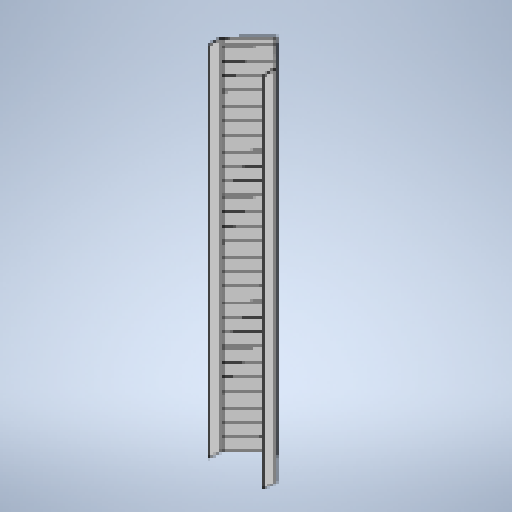
# Autodesk Inventor part: DSB-514 roof 4
Saved by Autodesk Inventor 2025 (Build 290162010, 162A)
## iProperties
Created: 2024-07-24
Part Number: DSB-514 roof 4
Material: Stainless Steel
Document SubType Name: Sheet Metal
Designer: admin
Density: 8 g/cm^3
Flat Pattern Width: 7.85084 cm
Flat Pattern Length: 27.5 cm
Flat Pattern Area: 215.898 cm^2
Sheet Metal Rule: Default
Sheet Metal Width: 78,508 mm
Sheet Metal Length: 275,000 mm
Sheet Metal Area: 21589,801 mm^2
Appearance: Default
Author: admin
Autodesk Inventor part; units mm, degrees
note: some values were not read from the file. Chosen so that the rebuilt part matches the saved one: flange form of "Plate1".
ref_plane "YZ Plane" through (0, 0, 0) normal (1, 0, 0) x (0, 1, 0)
ref_plane "XZ Plane" through (0, 0, 0) normal (0, 1, 0) x (-1, 0, 0)
ref_plane "XY Plane" through (0, 0, 0) normal (0, 0, 1) x (1, 0, 0)
sketch "Sketch3" plane through (0, 0, 0) normal (0, 0, 1) x (1, 0, 0)
  line L0 (-21, -10) -> (-21, -0.404026)
  line L1 (-21, 0) -> (-20.71934, 0.290632) construction
  line L2 (0, 21.746137) -> (0.71934, 21.001238) construction
  line L3 (21, 0) -> (21, -0.404026) construction
  line L4 (0, 21.746137) -> (0, 0) construction
  arc A0 (0.71934, 21.001238) -> (-0.71934, 21.001238) centre (0, 20.30658) ccw
  arc A1 (-20.71934, 0.290632) -> (-21, -0.404026) centre (-20, -0.404026) ccw
  arc A2 (21, -0.404026) -> (20.71934, 0.290632) centre (20, -0.404026) ccw
  line L5 (20.71934, 0.290632) -> (21, 0) construction
  line L6 (21, -0.404026) -> (21, -10)
  line L7 (-20.71934, 0.290632) -> (-0.71934, 21.001238)
  line L8 (-21, -0.404026) -> (-21, 0) construction
  line L9 (0.71934, 21.001238) -> (20.71934, 0.290632)
  line L10 (-0.71934, 21.001238) -> (0, 21.746137) construction
  dimension "d15" = 10
  dimension "d18" = 1
  dimension "d19" = 1
  dimension "d20" = 1
  dimension "d32" = 42
  dimension "d33" = 88
  measures "d15" distance of L3.start L6.end
  measures "d18" radius of A0
  measures "d19" radius of A1
  measures "d20" radius of A2
  measures "d32" distance between parallel lines of L6 L0
  measures "d33" angle of L9 L7
contour flange "Contour Flange1" sketch "Sketch3" thickness 0.8 bend radius 0.8 width 275 along (0, 0, -1) mid plane no both sides no wall seen from (-21, -5.202013, 0) lies toward (1, 0, 0) curves L0 A1 L7 A0 L9 A2 L6
bend "Bend1"
corner "Corner1"
sketch "Sketch5" plane through (20.71934, 0.290632, 0) normal (0.7193398, 0.6946584, 0) x (-0.6946584, 0.7193398, 0)
  line L0 (0, -275) -> (0, 0) construction
  line L1 (0, 0) -> (28.791131, 0) construction
  line L2 (28.791131, 0) -> (28.791131, -275) construction
  line L3 (28.791131, -275) -> (0, -275) construction
  line L4 (28.291131, -5.1) -> (0.291131, -5.1) construction
  line L5 (28.291131, -5) -> (0.291131, -5)
  line L6 (0.291131, -5.2) -> (28.291131, -5.2)
  arc A0 (28.291131, -5.2) -> (28.291131, -5) centre (28.291131, -5.1) ccw
  arc A1 (0.291131, -5) -> (0.291131, -5.2) centre (0.291131, -5.1) ccw
  line L7 (28.291131, -15.1) -> (0.291131, -15.1) construction
  line L8 (28.291131, -15) -> (0.291131, -15)
  line L9 (0.291131, -15.2) -> (28.291131, -15.2)
  arc A2 (28.291131, -15.2) -> (28.291131, -15) centre (28.291131, -15.1) ccw
  arc A3 (0.291131, -15) -> (0.291131, -15.2) centre (0.291131, -15.1) ccw
  line L10 (28.291131, -25.1) -> (0.291131, -25.1) construction
  line L11 (28.291131, -25) -> (0.291131, -25)
  line L12 (0.291131, -25.2) -> (28.291131, -25.2)
  arc A4 (28.291131, -25.2) -> (28.291131, -25) centre (28.291131, -25.1) ccw
  arc A5 (0.291131, -25) -> (0.291131, -25.2) centre (0.291131, -25.1) ccw
  line L13 (28.291131, -35.1) -> (0.291131, -35.1) construction
  line L14 (28.291131, -35) -> (0.291131, -35)
  line L15 (0.291131, -35.2) -> (28.291131, -35.2)
  arc A6 (28.291131, -35.2) -> (28.291131, -35) centre (28.291131, -35.1) ccw
  arc A7 (0.291131, -35) -> (0.291131, -35.2) centre (0.291131, -35.1) ccw
  line L16 (28.291131, -45.1) -> (0.291131, -45.1) construction
  line L17 (28.291131, -45) -> (0.291131, -45)
  line L18 (0.291131, -45.2) -> (28.291131, -45.2)
  arc A8 (28.291131, -45.2) -> (28.291131, -45) centre (28.291131, -45.1) ccw
  arc A9 (0.291131, -45) -> (0.291131, -45.2) centre (0.291131, -45.1) ccw
  line L19 (28.291131, -55.1) -> (0.291131, -55.1) construction
  line L20 (28.291131, -55) -> (0.291131, -55)
  line L21 (0.291131, -55.2) -> (28.291131, -55.2)
  arc A10 (28.291131, -55.2) -> (28.291131, -55) centre (28.291131, -55.1) ccw
  arc A11 (0.291131, -55) -> (0.291131, -55.2) centre (0.291131, -55.1) ccw
  line L22 (28.291131, -65.1) -> (0.291131, -65.1) construction
  line L23 (28.291131, -65) -> (0.291131, -65)
  line L24 (0.291131, -65.2) -> (28.291131, -65.2)
  arc A12 (28.291131, -65.2) -> (28.291131, -65) centre (28.291131, -65.1) ccw
  arc A13 (0.291131, -65) -> (0.291131, -65.2) centre (0.291131, -65.1) ccw
  line L25 (28.291131, -75.1) -> (0.291131, -75.1) construction
  line L26 (28.291131, -75) -> (0.291131, -75)
  line L27 (0.291131, -75.2) -> (28.291131, -75.2)
  arc A14 (28.291131, -75.2) -> (28.291131, -75) centre (28.291131, -75.1) ccw
  arc A15 (0.291131, -75) -> (0.291131, -75.2) centre (0.291131, -75.1) ccw
  line L28 (28.291131, -85.1) -> (0.291131, -85.1) construction
  line L29 (28.291131, -85) -> (0.291131, -85)
  line L30 (0.291131, -85.2) -> (28.291131, -85.2)
  arc A16 (28.291131, -85.2) -> (28.291131, -85) centre (28.291131, -85.1) ccw
  arc A17 (0.291131, -85) -> (0.291131, -85.2) centre (0.291131, -85.1) ccw
  line L31 (28.291131, -95.1) -> (0.291131, -95.1) construction
  line L32 (28.291131, -95) -> (0.291131, -95)
  line L33 (0.291131, -95.2) -> (28.291131, -95.2)
  arc A18 (28.291131, -95.2) -> (28.291131, -95) centre (28.291131, -95.1) ccw
  arc A19 (0.291131, -95) -> (0.291131, -95.2) centre (0.291131, -95.1) ccw
  line L34 (28.291131, -105.1) -> (0.291131, -105.1) construction
  line L35 (28.291131, -105) -> (0.291131, -105)
  line L36 (0.291131, -105.2) -> (28.291131, -105.2)
  arc A20 (28.291131, -105.2) -> (28.291131, -105) centre (28.291131, -105.1) ccw
  arc A21 (0.291131, -105) -> (0.291131, -105.2) centre (0.291131, -105.1) ccw
  line L37 (28.291131, -115.1) -> (0.291131, -115.1) construction
  line L38 (28.291131, -115) -> (0.291131, -115)
  line L39 (0.291131, -115.2) -> (28.291131, -115.2)
  arc A22 (28.291131, -115.2) -> (28.291131, -115) centre (28.291131, -115.1) ccw
  arc A23 (0.291131, -115) -> (0.291131, -115.2) centre (0.291131, -115.1) ccw
  line L40 (28.291131, -125.1) -> (0.291131, -125.1) construction
  line L41 (28.291131, -125) -> (0.291131, -125)
  line L42 (0.291131, -125.2) -> (28.291131, -125.2)
  arc A24 (28.291131, -125.2) -> (28.291131, -125) centre (28.291131, -125.1) ccw
  arc A25 (0.291131, -125) -> (0.291131, -125.2) centre (0.291131, -125.1) ccw
  line L43 (28.291131, -135.1) -> (0.291131, -135.1) construction
  line L44 (28.291131, -135) -> (0.291131, -135)
  line L45 (0.291131, -135.2) -> (28.291131, -135.2)
  arc A26 (28.291131, -135.2) -> (28.291131, -135) centre (28.291131, -135.1) ccw
  arc A27 (0.291131, -135) -> (0.291131, -135.2) centre (0.291131, -135.1) ccw
  line L46 (28.291131, -145.1) -> (0.291131, -145.1) construction
  line L47 (28.291131, -145) -> (0.291131, -145)
  line L48 (0.291131, -145.2) -> (28.291131, -145.2)
  arc A28 (28.291131, -145.2) -> (28.291131, -145) centre (28.291131, -145.1) ccw
  arc A29 (0.291131, -145) -> (0.291131, -145.2) centre (0.291131, -145.1) ccw
  line L49 (28.291131, -155.1) -> (0.291131, -155.1) construction
  line L50 (28.291131, -155) -> (0.291131, -155)
  line L51 (0.291131, -155.2) -> (28.291131, -155.2)
  arc A30 (28.291131, -155.2) -> (28.291131, -155) centre (28.291131, -155.1) ccw
  arc A31 (0.291131, -155) -> (0.291131, -155.2) centre (0.291131, -155.1) ccw
  line L52 (28.291131, -165.1) -> (0.291131, -165.1) construction
  line L53 (28.291131, -165) -> (0.291131, -165)
  line L54 (0.291131, -165.2) -> (28.291131, -165.2)
  arc A32 (28.291131, -165.2) -> (28.291131, -165) centre (28.291131, -165.1) ccw
  arc A33 (0.291131, -165) -> (0.291131, -165.2) centre (0.291131, -165.1) ccw
  line L55 (28.291131, -175.1) -> (0.291131, -175.1) construction
  line L56 (28.291131, -175) -> (0.291131, -175)
  line L57 (0.291131, -175.2) -> (28.291131, -175.2)
  arc A34 (28.291131, -175.2) -> (28.291131, -175) centre (28.291131, -175.1) ccw
  arc A35 (0.291131, -175) -> (0.291131, -175.2) centre (0.291131, -175.1) ccw
  line L58 (28.291131, -185.1) -> (0.291131, -185.1) construction
  line L59 (28.291131, -185) -> (0.291131, -185)
  line L60 (0.291131, -185.2) -> (28.291131, -185.2)
  arc A36 (28.291131, -185.2) -> (28.291131, -185) centre (28.291131, -185.1) ccw
  arc A37 (0.291131, -185) -> (0.291131, -185.2) centre (0.291131, -185.1) ccw
  line L61 (28.291131, -195.1) -> (0.291131, -195.1) construction
  line L62 (28.291131, -195) -> (0.291131, -195)
  line L63 (0.291131, -195.2) -> (28.291131, -195.2)
  arc A38 (28.291131, -195.2) -> (28.291131, -195) centre (28.291131, -195.1) ccw
  arc A39 (0.291131, -195) -> (0.291131, -195.2) centre (0.291131, -195.1) ccw
  line L64 (28.291131, -205.1) -> (0.291131, -205.1) construction
  line L65 (28.291131, -205) -> (0.291131, -205)
  line L66 (0.291131, -205.2) -> (28.291131, -205.2)
  arc A40 (28.291131, -205.2) -> (28.291131, -205) centre (28.291131, -205.1) ccw
  arc A41 (0.291131, -205) -> (0.291131, -205.2) centre (0.291131, -205.1) ccw
  line L67 (28.291131, -215.1) -> (0.291131, -215.1) construction
  line L68 (28.291131, -215) -> (0.291131, -215)
  line L69 (0.291131, -215.2) -> (28.291131, -215.2)
  arc A42 (28.291131, -215.2) -> (28.291131, -215) centre (28.291131, -215.1) ccw
  arc A43 (0.291131, -215) -> (0.291131, -215.2) centre (0.291131, -215.1) ccw
  line L70 (28.291131, -225.1) -> (0.291131, -225.1) construction
  line L71 (28.291131, -225) -> (0.291131, -225)
  line L72 (0.291131, -225.2) -> (28.291131, -225.2)
  arc A44 (28.291131, -225.2) -> (28.291131, -225) centre (28.291131, -225.1) ccw
  arc A45 (0.291131, -225) -> (0.291131, -225.2) centre (0.291131, -225.1) ccw
  line L73 (28.291131, -235.1) -> (0.291131, -235.1) construction
  line L74 (28.291131, -235) -> (0.291131, -235)
  line L75 (0.291131, -235.2) -> (28.291131, -235.2)
  arc A46 (28.291131, -235.2) -> (28.291131, -235) centre (28.291131, -235.1) ccw
  arc A47 (0.291131, -235) -> (0.291131, -235.2) centre (0.291131, -235.1) ccw
  line L76 (28.291131, -245.1) -> (0.291131, -245.1) construction
  line L77 (28.291131, -245) -> (0.291131, -245)
  line L78 (0.291131, -245.2) -> (28.291131, -245.2)
  arc A48 (28.291131, -245.2) -> (28.291131, -245) centre (28.291131, -245.1) ccw
  arc A49 (0.291131, -245) -> (0.291131, -245.2) centre (0.291131, -245.1) ccw
  line L79 (28.291131, -255.1) -> (0.291131, -255.1) construction
  line L80 (28.291131, -255) -> (0.291131, -255)
  line L81 (0.291131, -255.2) -> (28.291131, -255.2)
  arc A50 (28.291131, -255.2) -> (28.291131, -255) centre (28.291131, -255.1) ccw
  arc A51 (0.291131, -255) -> (0.291131, -255.2) centre (0.291131, -255.1) ccw
  line L82 (28.291131, -265.1) -> (0.291131, -265.1) construction
  line L83 (28.291131, -265) -> (0.291131, -265)
  line L84 (0.291131, -265.2) -> (28.291131, -265.2)
  arc A52 (28.291131, -265.2) -> (28.291131, -265) centre (28.291131, -265.1) ccw
  arc A53 (0.291131, -265) -> (0.291131, -265.2) centre (0.291131, -265.1) ccw
  point P0 (14.1838, 0)
  point P1 (14.291131, -5.1)
  point P2 (14.291131, -15.1)
  point P3 (14.291131, -25.1)
  point P4 (14.291131, -35.1)
  point P5 (14.291131, -45.1)
  point P6 (14.291131, -55.1)
  point P7 (14.291131, -65.1)
  point P8 (14.291131, -75.1)
  point P9 (14.291131, -85.1)
  point P10 (14.291131, -95.1)
  point P11 (14.291131, -105.1)
  point P12 (14.291131, -115.1)
  point P13 (14.291131, -125.1)
  point P14 (14.291131, -135.1)
  point P15 (14.291131, -145.1)
  point P16 (14.291131, -155.1)
  point P17 (14.291131, -165.1)
  point P18 (14.291131, -175.1)
  point P19 (14.291131, -185.1)
  point P20 (14.291131, -195.1)
  point P21 (14.291131, -205.1)
  point P22 (14.291131, -215.1)
  point P23 (14.291131, -225.1)
  point P24 (14.291131, -235.1)
  point P25 (14.291131, -245.1)
  point P26 (14.291131, -255.1)
  point P27 (14.291131, -265.1)
  dimension "d111" = 0.2
  dimension "d112" = 28
  dimension "d114" = 0.5
  dimension "d116" = 10
  dimension "d97" = 5
  constraints: 218 end point, 108 point on circle, 54 centre point, 4 tangent, 2 parallel, 1 midpoint, 1 perpendicular, 1 vertical, 312 other
  measures "d111" diameter of A1
  measures "d112" distance of L4.start L4.end
  measures "d114" distance from line of L4.start L2
  measures "d116" distance of L5.start L8.start
  measures "d97" distance between parallel lines of L5 L1
extrude "Cut3" cut sketch "Sketch5" against normal blind 0.8
mirror "Mirror2" about plane through (0, 0, 0) normal (1, 0, 0) of "Cut3"
sketch "Sketch9" plane through (0, 0, 0) normal (1, 0, 0) x (0, 1, 0)
  line L0 (-0.404026, -275) -> (-0.265095, -275)
  line L1 (21.001238, -275) -> (0.290632, -275)
  line L2 (-0.265095, -275) -> (0.290632, -275)
  line L3 (-0.404026, -275) -> (0.290632, -275)
  line L4 (-0.404026, -275) -> (-10, -275)
  line L5 (-0.404026, -275) -> (-10, -275)
  line L6 (-0.404026, -275) -> (0.290632, -275)
  line L7 (-10, -275) -> (-0.404026, -275)
  line L8 (-10, -275) -> (-0.404026, -275)
  line L9 (-0.404026, -275) -> (-0.265095, -275)
  line L10 (-0.265095, -275) -> (0.290632, -275)
  line L11 (21.001238, -275) -> (21.30658, -275)
  line L12 (-0.265095, -275) -> (20.445512, -275)
  line L13 (20.445512, -275) -> (21.001238, -275)
  line L14 (0.290632, -275) -> (21.001238, -275)
  line L15 (20.445512, -275) -> (20.50658, -275)
  line L16 (20.445512, -275) -> (-0.265095, -275)
  line L17 (20.445512, -275) -> (21.001238, -275)
  line L18 (-0.265095, -275) -> (0.290632, -275)
  line L19 (-0.404026, -275) -> (-0.265095, -275)
  line L20 (-0.404026, -275) -> (0.290632, -275)
  line L21 (20.445512, -275) -> (21.001238, -275)
  line L22 (20.445512, -275) -> (20.445512, -275)
  line L23 (20.445512, -275) -> (21.001238, -275)
  line L24 (21.001238, -275) -> (21.001238, -275)
  line L25 (-0.265095, -275) -> (0.290632, -275)
  line L26 (20.445512, -275) -> (-0.265095, -275)
  line L27 (20.445512, -275) -> (21.001238, -275)
  line L28 (21.001238, -275) -> (0.290632, -275)
  line L29 (20.445512, -275) -> (21.001238, -275)
  line L30 (-0.265095, -275) -> (20.445512, -275)
  line L31 (-0.265095, -275) -> (0.290632, -275)
  line L32 (0.290632, -275) -> (21.001238, -275)
  line L33 (-10, -275) -> (-0.404026, -275)
  line L34 (-10, -275) -> (-0.404026, -275)
  line L35 (-0.265095, -275) -> (-0.404026, -275)
  line L36 (-0.265095, -275) -> (0.290632, -275)
  line L37 (0.290632, -275) -> (-0.404026, -275)
  line L38 (-0.404026, -275) -> (-10, -275)
  line L39 (-0.404026, -275) -> (-10, -275)
  line L40 (-10, 0) -> (-10, -275)
  line L41 (-10, -273.934687) -> (20.50658, -275)
  point P0 (0, 0)
extrude "Extrusion4" cut sketch "Sketch9" along normal through all both and the other way through all
equation "\"d21\" = Thickness"
equation "\"d22\" = BendReliefWidth"
equation "\"d23\" = BendReliefDepth"
equation "\"d24\" = MinimumRemnant"
equation "\"d25\" = TransitionRadius"
equation "\"d27\" = BendRadius"
equation "\"d29\" = CornerReliefSize"
equation "\"d30\" = GapSize"
equation "\"d31\" = JacobiRadiusSize"
equation "\"BendRadius\" = Thickness"
equation "\"BendReliefWidth\" = Thickness"
equation "\"BendReliefDepth\" = 0.5 * Thickness"
equation "\"CornerReliefSize\" = 4 * Thickness"
equation "\"MinimumRemnant\" = 2 * Thickness"
equation "\"TransitionRadius\" = BendRadius"
equation "\"JacobiRadiusSize\" = BendRadius"
equation "\"GapSize\" = Thickness"
equation "\"grat_thick\" = 0.2"
equation "\"grat_lenth\" = 28"
equation "\"grat_indet_X\" = 5"
equation "\"grat_indet_Y\" = 0.5"
equation "\"Thickness\" = 0.8"
body "Solid2"
